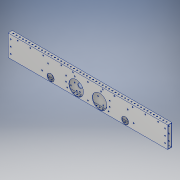
# Autodesk Inventor part: Side Extrusion
Saved by Autodesk Inventor 2019.4 (Build 234330000, 330)
## iProperties
Created: 2019-11-02
Part Number: Side Extrusion
Material: Aluminum 6061
Document SubType Name: Modeling
Designer: admin
Density: 2.7 g/cm^3
Appearance: Aluminum - Flat
Mass: 868.057 g
Surface Area: 3271.09 cm^2
Volume: 321.503 cm^3
Author: admin
Autodesk Inventor part; units mm, degrees
ref_plane "YZ Plane" through (0, 0, 0) normal (1, 0, 0) x (0, 1, 0)
ref_plane "XZ Plane" through (0, 0, 0) normal (0, 1, 0) x (-1, 0, 0)
ref_plane "XY Plane" through (0, 0, 0) normal (0, 0, 1) x (1, 0, 0)
sketch "Sketch1" plane through (0, 0, 0) normal (1, 0, 0) x (0, 1, 0)
  line L0 (-50, 10) -> (50, 10)
  line L1 (50, 10) -> (50, -10)
  line L2 (50, -10) -> (-50, -10)
  line L3 (-50, -10) -> (-50, 10)
  line L4 (-50, 10) -> (50, -10) construction
  line L5 (50, 10) -> (-50, -10) construction
  line L6 (48, -8) -> (48, 8)
  line L7 (48, 8) -> (-48, 8)
  line L8 (-48, 8) -> (-48, -8)
  line L9 (-48, -8) -> (48, -8)
  point P0 (0, 0)
  dimension "d0" = 100
  dimension "d1" = 20
  dimension "d2" = 2
  constraints: 20 end point, 4 parallel, 2 midpoint, 2 perpendicular, 1 horizontal, 3 other
  measures "d0" distance of L1.end L2.end
  measures "d1" distance of L0.end L1.end
  measures "d2" distance between parallel lines of L1 L6
extrude "Extrusion1" add sketch "Sketch1" along normal blind 750
sketch "Sketch2" plane through (0, -50, 10) normal (0, 0, -1) x (-1, 0, 0)
  circle A0 centre (-200, 18.3) radius 16.3
  line L0 (0, 0) -> (-750, 0) projected
  line L1 (0, 100) -> (0, 0) projected
  line L2 (0, 100) -> (-750, 100) projected
  line L3 (-375, 100) -> (-375, 0)
  line L4 (0, 0) -> (-750, 0) projected
  circle A1 centre (-550, 18.3) radius 16.3
  point P0 (0, 50)
  dimension "d5" = 32.6
  dimension "d6" = 18.3
  dimension "d9" = 200
  constraints: 2 centre point, 2 end point, 2 midpoint, 1 symmetric about line, 1 other
  measures "d5" diameter of A0
  measures "d6" distance from line of L0 A0.centre
  measures "d9" distance from line of L1 A0.centre
extrude "Extrusion2" cut sketch "Sketch2" along normal blind 2 contours A0 | A1
sketch "Sketch3" plane through (0, -50, 10) normal (0, 0, 1) x (1, 0, 0)
  circle A0 centre (320, 36) radius 34
  line L0 (0, 0) -> (0, 100) projected
  line L1 (0, 0) -> (750, 0) projected
  line L2 (375, 100) -> (375, 0)
  circle A1 centre (430, 36) radius 34
  point P0 (0, 50)
  dimension "d10" = 68
  dimension "d11" = 320
  dimension "d12" = 36
  constraints: 2 centre point, 2 end point, 1 midpoint, 1 symmetric about line, 1 other
  measures "d10" diameter of A0
  measures "d11" distance from line of L0 A0.centre
  measures "d12" distance from line of A0.centre L1
extrude "Extrusion3" cut sketch "Sketch3" against normal blind 2
sketch "Sketch4" plane through (0, -50, -10) normal (0, 0, -1) x (-1, 0, 0)
  circle A0 centre (-200, 18.3) radius 16.3 construction
  circle A1 centre (-200, 18.3) radius 16.3 construction
  circle A2 centre (-200, 18.3) radius 12.3
  line L0 (0, 0) -> (-750, 0) projected
  line L1 (-375, 0) -> (-375, 100)
  line L2 (0, 100) -> (-750, 100) projected
  circle A3 centre (-550, 18.3) radius 12.3
  point P0 (0, 50)
  point P1 (-200, 2)
  dimension "d17" = 24.6
  constraints: 2 centre point, 2 end point, 2 midpoint, 1 coincident, 1 symmetric about line, 1 vertical alignment, 1 other
  measures "d17" diameter of A2
extrude "Extrusion4" cut sketch "Sketch4" against normal blind 2
sketch "Sketch5" plane through (0, -50, -10) normal (0, 0, -1) x (-1, 0, 0)
  circle A0 centre (-216, 18.3) radius 2.25
  circle A1 centre (-200, 18.3) radius 12.3 projected
  line L0 (-200, 18.3) -> (-216, 18.3) construction
  circle A2 centre (-200, 34.3) radius 2.25
  circle A3 centre (-184, 18.3) radius 2.25
  line L1 (0, 100) -> (-750, 100) projected
  line L2 (-375, 100) -> (-375, 0)
  line L3 (0, 0) -> (-750, 0) projected
  circle A4 centre (-534, 18.3) radius 2.25
  circle A5 centre (-550, 34.3) radius 2.25
  circle A6 centre (-566, 18.3) radius 2.25
  point P0 (0, 50)
  dimension "d18" = 4.5
  dimension "d21" = 16
  dimension "d24" = 180
  constraints: 6 centre point, 4 end point, 3 symmetric about line, 2 midpoint, 1 horizontal, 8 other
  measures "d18" diameter of A0
  measures "d21" distance of L0.start L0.end
extrude "Extrusion5" cut sketch "Sketch5" against normal blind 2 contours A0 | A2 | A3 | A4 | A5 | A6
sketch "Sketch6" plane through (0, -50, -10) normal (0, 0, -1) x (-1, 0, 0)
  circle A0 centre (-320, 36) radius 10
  line L0 (0, 0) -> (-750, 0)
  line L1 (0, 100) -> (0, 0)
  circle A1 centre (-320, 36) radius 25.4
  circle A2 centre (-320, 61.4) radius 2.75
  circle A3 centre (-345.4, 36) radius 2.75
  circle A4 centre (-320, 10.6) radius 2.75
  circle A5 centre (-294.6, 36) radius 2.75
  line L2 (-253.017411, 23.435515) -> (-232.892456, 42.298093)
  arc A6 (-232.892456, 42.298093) -> (-221.757712, 42.917915) centre (-228.087048, 56.296238) ccw
  line L3 (-221.757712, 42.917915) -> (-214.444374, 31.843064)
  arc A7 (-214.444374, 31.843064) -> (-219.510833, 21.673419) centre (-200.000281, 18.300238) ccw
  line L4 (-219.510833, 21.673419) -> (-250.639269, 18.264485)
  arc A8 (-253.017411, 23.435515) -> (-250.639269, 18.264485) centre (-250.965852, 21.246656) ccw
  line L5 (-211.270738, 53.460853) -> (-194.873773, 53.460853)
  arc A9 (-192.370354, 52.113999) -> (-194.873773, 53.460853) centre (-194.873773, 50.460853) ccw
  line L6 (-192.370354, 52.113999) -> (-179.138455, 32.076457)
  arc A10 (-175.03962, 16.898311) -> (-179.138455, 32.076457) centre (-200.000281, 18.300238) ccw
  arc A11 (-178.034899, 14.066542) -> (-175.03962, 16.898311) centre (-178.034899, 17.066542) ccw
  arc A12 (-180.234557, 17.135693) -> (-178.034899, 14.066542) centre (-177.23975, 16.959247) ccw
  arc A13 (-180.234557, 17.135693) -> (-207.163495, 36.759066) centre (-200.000281, 18.300238) ccw
  arc A14 (-210.67628, 37.793051) -> (-207.163495, 36.759066) centre (-208.248831, 39.555859) ccw
  line L7 (-210.67628, 37.793051) -> (-215.684337, 44.689327)
  arc A15 (-215.756353, 48.111253) -> (-215.684337, 44.689327) centre (-213.256888, 46.452134) ccw
  arc A16 (-215.756353, 48.111253) -> (-214.104947, 51.444344) centre (-228.087048, 56.296238) ccw
  arc A17 (-211.270738, 53.460853) -> (-214.104947, 51.444344) centre (-211.270738, 50.460853) ccw
  line L8 (-284.564398, 40.381936) -> (-284.260118, 32.912505)
  arc A18 (-288.469729, 30.046162) -> (-284.260118, 32.912505) centre (-287.257632, 32.790396) ccw
  line L9 (-288.469729, 30.046162) -> (-290.947938, 31.140759)
  arc A19 (-305.775526, 47.161395) -> (-290.947938, 31.140759) centre (-279.837048, 56.296238) ccw
  arc A20 (-302.945874, 51.157924) -> (-305.775526, 47.161395) centre (-302.945874, 48.157924) ccw
  line L10 (-302.945874, 51.157924) -> (-295.667646, 51.157924)
  arc A21 (-292.999568, 49.529549) -> (-295.667646, 51.157924) centre (-295.667646, 48.157924) ccw
  arc A22 (-292.999568, 49.529549) -> (-286.259969, 42.962593) centre (-279.837048, 56.296238) ccw
  arc A23 (-284.564398, 40.381936) -> (-286.259969, 42.962593) centre (-287.561912, 40.259827) ccw
  arc A24 (-215.577348, -2.149578) -> (-212.475123, 2.924338) centre (-214.365251, 0.594656) ccw
  line L11 (-215.577348, -2.149578) -> (-233.291666, 5.674635)
  arc A25 (-232.501757, 11.389014) -> (-233.291666, 5.674635) centre (-232.079569, 8.418869) ccw
  line L12 (-232.501757, 11.389014) -> (-221.643204, 12.932492)
  arc A26 (-218.428814, 11.059438) -> (-221.643204, 12.932492) centre (-221.221015, 9.962348) ccw
  arc A27 (-218.428814, 11.059438) -> (-212.475123, 2.924338) centre (-200.000281, 18.300238) ccw
  line L13 (-193.41702, -3.03817) -> (-193.41702, -1.738915)
  arc A28 (-192.204475, 0.099539) -> (-193.41702, -1.738915) centre (-191.41702, -1.738915) ccw
  arc A29 (-192.204475, 0.099539) -> (-186.247248, 4.056148) centre (-200.000281, 18.300238) ccw
  arc A30 (-184.858053, 4.617351) -> (-186.247248, 4.056148) centre (-184.858053, 2.617351) ccw
  line L14 (-184.858053, 4.617351) -> (-183.176278, 4.617351)
  arc A31 (-181.713321, 1.253622) -> (-183.176278, 4.617351) centre (-183.176278, 2.617351) ccw
  arc A32 (-190.67065, -4.893684) -> (-181.713321, 1.253622) centre (-200.000281, 18.300238) ccw
  arc A33 (-193.41702, -3.03817) -> (-190.67065, -4.893684) centre (-191.41702, -3.03817) ccw
  line L15 (-284.642456, 79.519622) -> (-284.642456, 72.2936)
  arc A34 (-286.326938, 69.597415) -> (-284.642456, 72.2936) centre (-287.642456, 72.2936) ccw
  arc A35 (-286.326938, 69.597415) -> (-292.999568, 63.062926) centre (-279.837048, 56.296238) ccw
  arc A36 (-295.667646, 61.434552) -> (-292.999568, 63.062926) centre (-295.667646, 64.434552) ccw
  line L16 (-295.667646, 61.434552) -> (-302.945874, 61.434552)
  arc A37 (-305.775526, 65.43108) -> (-302.945874, 61.434552) centre (-302.945874, 64.434552) ccw
  arc A38 (-288.598221, 82.363302) -> (-305.775526, 65.43108) centre (-279.837048, 56.296238) ccw
  arc A39 (-284.642456, 79.519622) -> (-288.598221, 82.363302) centre (-287.642456, 79.519622) ccw
  line L17 (-228.549746, 83.796238) -> (-228.087048, 83.796238)
  arc A40 (-205.139039, 71.450079) -> (-228.087048, 83.796238) centre (-228.087048, 56.296238) ccw
  line L18 (-205.139039, 71.450079) -> (-200.07721, 63.784769)
  arc A41 (-202.580629, 59.131623) -> (-200.07721, 63.784769) centre (-202.580629, 62.131623) ccw
  line L19 (-202.580629, 59.131623) -> (-211.270738, 59.131623)
  arc A42 (-214.104947, 61.148131) -> (-211.270738, 59.131623) centre (-211.270738, 62.131623) ccw
  arc A43 (-214.104947, 61.148131) -> (-226.324022, 70.990854) centre (-228.087048, 56.296238) ccw
  arc A44 (-228.77251, 72.907815) -> (-226.324022, 70.990854) centre (-225.966651, 73.969492) ccw
  line L20 (-228.77251, 72.907815) -> (-231.355605, 79.734561)
  arc A45 (-228.549746, 83.796238) -> (-231.355605, 79.734561) centre (-228.549746, 80.796238) ccw
  line L21 (-265.557874, 52.404554) -> (-242.366221, 52.404554)
  arc A46 (-242.366221, 52.404554) -> (-238.505976, 45.785009) centre (-228.087048, 56.296238) ccw
  line L22 (-238.505976, 45.785009) -> (-267.245911, 24.914144)
  arc A47 (-271.925902, 26.641566) -> (-267.245911, 24.914144) centre (-269.008718, 27.341593) ccw
  line L23 (-271.925902, 26.641566) -> (-275.026214, 39.561319)
  arc A48 (-273.411505, 42.963856) -> (-275.026214, 39.561319) centre (-272.10903, 40.261346) ccw
  arc A49 (-273.411505, 42.963856) -> (-265.557874, 52.404554) centre (-279.837048, 56.296238) ccw
  line L24 (-244.498772, 60.187921) -> (-263.425323, 60.187921)
  arc A50 (-266.191344, 62.026401) -> (-263.425323, 60.187921) centre (-263.425323, 63.187921) ccw
  arc A51 (-266.191344, 62.026401) -> (-271.308518, 68.391864) centre (-279.837048, 56.296238) ccw
  arc A52 (-272.579762, 70.843681) -> (-271.308518, 68.391864) centre (-269.579762, 70.843681) ccw
  line L25 (-272.579762, 70.843681) -> (-272.579762, 80.796238)
  arc A53 (-269.579762, 83.796238) -> (-272.579762, 80.796238) centre (-269.579762, 80.796238) ccw
  line L26 (-269.579762, 83.796238) -> (-241.985589, 83.796238)
  arc A54 (-239.347045, 82.223854) -> (-241.985589, 83.796238) centre (-241.985589, 80.796238) ccw
  line L27 (-239.347045, 82.223854) -> (-234.411772, 73.102405)
  arc A55 (-235.539652, 69.082898) -> (-234.411772, 73.102405) centre (-237.050316, 71.674789) ccw
  arc A56 (-235.539652, 69.082898) -> (-241.732751, 62.026401) centre (-228.087048, 56.296238) ccw
  arc A57 (-244.498772, 60.187921) -> (-241.732751, 62.026401) centre (-244.498772, 63.187921) ccw
  circle A58 centre (-188.087048, 69.219011) radius 2.75
  circle A59 centre (-277.837048, 16.582771) radius 2.75
  circle A60 centre (-250.087048, 92.776028) radius 2.75
  circle A61 centre (-160.000311, 27.300374) radius 2.75
  circle A62 centre (-313.422281, 79.812871) radius 2.75
  circle A63 centre (-200.000281, 18.300238) radius 9.8
  circle A64 centre (-228.087048, 56.296238) radius 9.8
  circle A65 centre (-279.837048, 56.296238) radius 9.8
  arc A66 (-244.094053, 93.065883) -> (-256.080042, 92.486173) centre (-250.087048, 92.776028) ccw
  line L28 (-256.080042, 92.486173) -> (-281.527869, 91.255373)
  arc A67 (-281.527869, 91.255373) -> (-302.063857, 83.332675) centre (-279.837048, 56.296238) ccw
  line L29 (-312.063857, 85.657072) -> (-302.063857, 83.332675)
  arc A68 (-312.063857, 85.657072) -> (-318.449425, 76.537536) centre (-313.422281, 79.812871) ccw
  line L30 (-312.845005, 67.9356) -> (-318.449425, 76.537536)
  arc A69 (-312.845005, 67.9356) -> (-294.877782, 24.692815) centre (-279.837048, 56.296238) ccw
  line L31 (-294.877782, 24.692815) -> (-283.254777, 19.161182)
  arc A70 (-283.254777, 19.161182) -> (-272.419318, 14.004359) centre (-277.837048, 16.582771) ccw
  line L32 (-272.419318, 14.004359) -> (-215.041015, -13.303185)
  arc A71 (-215.041015, -13.303185) -> (-165.129101, 21.300374) centre (-200.000281, 18.300238) ccw
  line L33 (-160.000311, 21.300374) -> (-165.129101, 21.300374)
  arc A72 (-160.000311, 21.300374) -> (-160.000311, 33.300374) centre (-160.000311, 27.300374) ccw
  line L34 (-168.377569, 33.300374) -> (-160.000311, 33.300374)
  arc A73 (-168.377569, 33.300374) -> (-170.793725, 37.586945) centre (-200.000281, 18.300238) ccw
  line L35 (-170.793725, 37.586945) -> (-187.727133, 63.229816)
  arc A74 (-187.727133, 63.229816) -> (-193.4538, 71.901914) centre (-188.087048, 69.219011) ccw
  line L36 (-193.4538, 71.901914) -> (-196.794309, 76.960567)
  arc A75 (-196.794309, 76.960567) -> (-229.898642, 93.752454) centre (-228.087048, 56.296238) ccw
  line L37 (-229.898642, 93.752454) -> (-244.094053, 93.065883)
  line L38 (0, 100) -> (-750, 100)
  line L39 (-375, 100) -> (-375, 0)
  circle A76 centre (-430, 61.4) radius 2.75
  circle A77 centre (-404.6, 36) radius 2.75
  circle A78 centre (-430, 10.6) radius 2.75
  circle A79 centre (-455.4, 36) radius 2.75
  circle A80 centre (-561.912952, 69.219011) radius 2.75
  circle A81 centre (-472.162952, 16.582771) radius 2.75
  circle A82 centre (-499.912952, 92.776028) radius 2.75
  circle A83 centre (-589.999689, 27.300374) radius 2.75
  circle A84 centre (-436.577719, 79.812871) radius 2.75
  point P0 (0, 50)
  dimension "d31" = 50.8
  dimension "d28" = 20
  dimension "d29" = 36
  dimension "d30" = 320
  dimension "d32" = 5.5
  dimension "d35" = 360
  dimension "d46" = 36
  constraints: 14 centre point, 9 symmetric about line, 2 end point, 2 midpoint, 1 coincident, 1 vertical alignment, 20 other
  measures "d28" diameter of A0
  measures "d29" distance from line of L0 A0.centre
  measures "d30" distance from line of L1 A0.centre
  measures "d32" diameter of A2
  measures "d46" distance from line of L0 A3.centre
extrude "Extrusion6" cut sketch "Sketch6" against normal blind 50 contours A0 | A2 A1 | A1 A2 | A4 A1 | A1 A4 | A5 A1 | A1 A5 A19 | A5 A19 | A3 A1 | A1 A3 | A58 | A59 | A60 | A61 | A62 | A76 | A77 | A78 | A79 | A80 | A81 | A82 | A83 | A84 picked at (-296.100043, 35.292413)
sketch "Sketch7" plane through (0, -50, -10) normal (0, 0, -1) x (-1, 0, 0)
  circle A0 centre (-228.087, 56.296) radius 10.5
  line L0 (0, 100) -> (-750, 100) projected
  line L1 (0, 100) -> (0, 0) projected
  circle A1 centre (-279.787, 56.296) radius 10.5
  line L2 (-228.087, 56.296) -> (-279.787, 56.296) construction
  line L3 (-375, 100) -> (-375, 0)
  circle A2 centre (-521.913, 56.296) radius 10.5
  circle A3 centre (-470.213, 56.296) radius 10.5
  point P0 (0, 50)
  dimension "d39" = 43.704
  dimension "d40" = 228.087
  dimension "d41" = 21
  dimension "d44" = 21
  dimension "d45" = 51.7
  constraints: 4 centre point, 4 end point, 2 symmetric about line, 1 horizontal, 1 midpoint, 1 vertical, 2 other
  measures "d39" distance from line of L0 L2.start
  measures "d40" distance from line of L1 L2.start
  measures "d41" diameter of A0
  measures "d44" diameter of A1
  measures "d45" distance of L2.start L2.end
extrude "Extrusion7" cut sketch "Sketch7" against normal up to surface (2 mm away)
sketch "Sketch8" plane through (0, -50, -10) normal (0, 0, -1) x (-1, 0, 0)
  circle A0 centre (-375, 87.5) radius 2.75
  circle A1 centre (-445, 92) radius 2.75
  circle A2 centre (-585, 90.5) radius 2.75
  circle A3 centre (-705, 90.5) radius 2.75
  circle A4 centre (-645, 90.5) radius 2.75
  circle A5 centre (-737.5, 50) radius 2.75
  circle A6 centre (-737.5, 80) radius 2.75
  circle A7 centre (-737.5, 20) radius 2.75
  circle A8 centre (-375, 12.5) radius 2.75
  circle A9 centre (-445, 8) radius 2.75
  line L0 (-750, 0) -> (-750, 100) construction
  line L1 (0, 100) -> (-750, 100) construction
  line L2 (0, 0) -> (-750, 0) construction
  line L3 (0, 0) -> (-750, 0)
  line L4 (-375, 0) -> (-375, 100)
  circle A10 centre (-305, 92) radius 2.75
  circle A11 centre (-165, 90.5) radius 2.75
  circle A12 centre (-45, 90.5) radius 2.75
  circle A13 centre (-105, 90.5) radius 2.75
  circle A14 centre (-12.5, 50) radius 2.75
  circle A15 centre (-12.5, 80) radius 2.75
  circle A16 centre (-12.5, 20) radius 2.75
  circle A17 centre (-305, 8) radius 2.75
  line L5 (0, 0) -> (0, 100) construction
  dimension "d49" = 5.5
  dimension "d50" = 5.5
  dimension "d51" = 5.5
  dimension "d52" = 12.5
  dimension "d53" = 12.5
  dimension "d54" = 12.5
  dimension "d55" = 20
  dimension "d56" = 20
  dimension "d57" = 50
  dimension "d58" = 45
  dimension "d59" = 105
  dimension "d60" = 60
  dimension "d61" = 9.5
  dimension "d62" = 9.5
  dimension "d63" = 9.5
  dimension "d64" = 5.5
  dimension "d65" = 5.5
  dimension "d66" = 5.5
  dimension "d80" = 12.5
  dimension "d81" = 8
  dimension "d84" = 8
  dimension "d88" = 305
  dimension "d89" = 305
  dimension "d90" = 12.5
  dimension "d91" = 100
  dimension "d92" = 750
  constraints: 18 centre point, 10 end point, 8 symmetric about line, 4 equal radius, 2 midpoint, 2 point on line, 8 other
  measures "d49" diameter of A6
  measures "d50" diameter of A5
  measures "d51" diameter of A7
  measures "d52" distance from line of L0 A7.centre
  measures "d53" distance from line of L0 A5.centre
  measures "d54" distance from line of L0 A6.centre
  measures "d55" distance from line of L1 A6.centre
  measures "d56" distance from line of L2 A7.centre
  measures "d57" distance from line of L1 A5.centre
  measures "d58" distance from line of L0 A3.centre
  measures "d59" distance from line of L0 A4.centre
  measures "d60" distance of A4.centre A2.centre
  measures "d61" distance from line of L1 A3.centre
  measures "d62" distance from line of L1 A4.centre
  measures "d63" distance from line of L1 A2.centre
  measures "d64" diameter of A3
  measures "d65" diameter of A4
  measures "d66" diameter of A2
  measures "d80" distance from line of L2 A8.centre
  measures "d81" distance from line of L2 A9.centre
  measures "d84" distance from line of L1 A1.centre
  measures "d88" distance from line of L0 A1.centre
  measures "d89" distance from line of L0 A9.centre
  measures "d90" distance from line of L1 A0.centre
  measures "d91" distance between parallel lines of L1 L3
  measures "d92" distance between parallel lines of L5 L0
extrude "Extrusion8" cut sketch "Sketch8" against normal blind 50
sketch "Sketch9" plane through (0, -50, 10) normal (0, 0, 1) x (1, 0, 0)
  circle A0 centre (272.5, 62.5) radius 2.75
  circle A1 centre (272.5, 37.5) radius 2.75
  line L0 (0, 100) -> (750, 100) projected
  line L1 (375, 100) -> (375, 0)
  line L2 (0, 0) -> (750, 0) projected
  line L3 (0, 0) -> (0, 100) projected
  circle A2 centre (477.5, 62.5) radius 2.75
  circle A3 centre (477.5, 37.5) radius 2.75
  point P0 (0, 50)
  dimension "d94" = 5.5
  dimension "d95" = 5.5
  dimension "d96" = 272.5
  dimension "d97" = 272.5
  dimension "d98" = 37.5
  dimension "d99" = 37.5
  constraints: 4 centre point, 2 end point, 2 midpoint, 2 symmetric about line, 2 other
  measures "d94" diameter of A0
  measures "d95" diameter of A1
  measures "d96" distance from line of L3 A0.centre
  measures "d97" distance from line of L3 A1.centre
  measures "d98" distance from line of L2 A1.centre
  measures "d99" distance from line of L0 A0.centre
extrude "Extrusion9" cut sketch "Sketch9" against normal blind 5 contours A0 | A1 | A2 | A3
sketch "Sketch10" plane through (0, 50, 10) normal (0, 1, 0) x (1, 0, 0)
  line L0 (0, 20) -> (750, 20) projected
  circle A0 centre (15, 10) radius 2.75
  line L1 (15, 10) -> (0, 10) construction
  circle A1 centre (30, 10) radius 2.75
  circle A2 centre (45, 10) radius 2.75
  circle A3 centre (60, 10) radius 2.75
  circle A4 centre (75, 10) radius 2.75
  circle A5 centre (90, 10) radius 2.75
  circle A6 centre (105, 10) radius 2.75
  circle A7 centre (120, 10) radius 2.75
  circle A8 centre (135, 10) radius 2.75
  circle A9 centre (150, 10) radius 2.75
  circle A10 centre (165, 10) radius 2.75
  circle A11 centre (180, 10) radius 2.75
  circle A12 centre (195, 10) radius 2.75
  circle A13 centre (210, 10) radius 2.75
  circle A14 centre (225, 10) radius 2.75
  circle A15 centre (240, 10) radius 2.75
  circle A16 centre (255, 10) radius 2.75
  circle A17 centre (270, 10) radius 2.75
  circle A18 centre (285, 10) radius 2.75
  circle A19 centre (300, 10) radius 2.75
  circle A20 centre (315, 10) radius 2.75
  circle A21 centre (330, 10) radius 2.75
  circle A22 centre (345, 10) radius 2.75
  circle A23 centre (360, 10) radius 2.75
  circle A24 centre (375, 10) radius 2.75
  circle A25 centre (390, 10) radius 2.75
  circle A26 centre (405, 10) radius 2.75
  circle A27 centre (420, 10) radius 2.75
  circle A28 centre (435, 10) radius 2.75
  circle A29 centre (450, 10) radius 2.75
  circle A30 centre (465, 10) radius 2.75
  circle A31 centre (480, 10) radius 2.75
  circle A32 centre (495, 10) radius 2.75
  circle A33 centre (510, 10) radius 2.75
  circle A34 centre (525, 10) radius 2.75
  circle A35 centre (540, 10) radius 2.75
  circle A36 centre (555, 10) radius 2.75
  circle A37 centre (570, 10) radius 2.75
  circle A38 centre (585, 10) radius 2.75
  circle A39 centre (600, 10) radius 2.75
  circle A40 centre (615, 10) radius 2.75
  circle A41 centre (630, 10) radius 2.75
  circle A42 centre (645, 10) radius 2.75
  circle A43 centre (660, 10) radius 2.75
  circle A44 centre (675, 10) radius 2.75
  circle A45 centre (690, 10) radius 2.75
  circle A46 centre (705, 10) radius 2.75
  circle A47 centre (720, 10) radius 2.75
  circle A48 centre (735, 10) radius 2.75
  dimension "d102" = 5.5
  dimension "d103" = 15
  dimension "d106" = 15
  constraints: 49 centre point, 2 end point, 2 horizontal, 96 other
  measures "d102" diameter of A0
  measures "d103" distance of L1.start L1.end
  measures "d106" distance of L1.start A1.centre
extrude "Extrusion10" cut sketch "Sketch10" against normal through all
equation "\"d97\" = d96"
equation "\"d98\" = d99"
body "Solid1"
